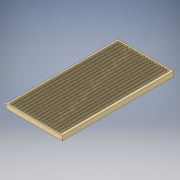
# Autodesk Inventor part: Lathhouse roof
Saved by Autodesk Inventor 2018 (Build 220112000, 112)
## iProperties
Created: 2019-05-09
Part Number: Lathhouse roof
Material: Generic
Document SubType Name: Modeling
Designer: 10043883
Density: 1 g/cm^3
Appearance: Wheat
Author: 10043883
Autodesk Inventor part; units mm, degrees
ref_plane "YZ Plane" through (0, 0, 0) normal (1, 0, 0) x (0, 1, 0)
ref_plane "XZ Plane" through (0, 0, 0) normal (0, 1, 0) x (-1, 0, 0)
ref_plane "XY Plane" through (0, 0, 0) normal (0, 0, 1) x (1, 0, 0)
sketch "Sketch1" plane through (0, 0, 0) normal (0, 1, 0) x (-1, 0, 0)
  line L0 (0, 0) -> (-3048, 0)
  line L1 (-3048, 0) -> (-3048, -6096)
  line L2 (-3048, -6096) -> (0, -6096)
  line L3 (0, -6096) -> (0, 0)
  dimension "d0" = 3048
  dimension "d1" = 6096
  constraints: 8 end point, 2 parallel, 1 horizontal, 1 perpendicular
  measures "d0" distance of L2.end L1.end
  measures "d1" distance of L1.end L0.end
extrude "Extrusion1" add sketch "Sketch1" along normal blind 254
sketch "Sketch2" plane through (0, 254, 0) normal (0, 1, 0) x (1, 0, 0)
  point P0 (0, 0)
sketch "Sketch3" plane through (0, 254, 0) normal (0, 1, 0) x (1, 0, 0)
  line L0 (94.7299, 6010.3245) -> (249.433, 6010.3245)
  line L1 (249.433, 6010.3245) -> (249.433, 63.9243)
  line L2 (249.433, 63.9243) -> (94.7299, 63.9243)
  line L3 (94.7299, 63.9243) -> (94.7299, 6010.3245)
  line L4 (427.233, 6010.3245) -> (427.233, 63.9243)
  line L5 (272.5299, 63.9243) -> (272.5299, 6010.3245)
  line L6 (427.233, 63.9243) -> (272.5299, 63.9243)
  line L7 (272.5299, 6010.3245) -> (427.233, 6010.3245)
  line L8 (605.033, 6010.3245) -> (605.033, 63.9243)
  line L9 (450.3299, 63.9243) -> (450.3299, 6010.3245)
  line L10 (605.033, 63.9243) -> (450.3299, 63.9243)
  line L11 (450.3299, 6010.3245) -> (605.033, 6010.3245)
  line L12 (782.833, 6010.3245) -> (782.833, 63.9243)
  line L13 (628.1299, 63.9243) -> (628.1299, 6010.3245)
  line L14 (782.833, 63.9243) -> (628.1299, 63.9243)
  line L15 (628.1299, 6010.3245) -> (782.833, 6010.3245)
  line L16 (960.633, 6010.3245) -> (960.633, 63.9243)
  line L17 (805.9299, 63.9243) -> (805.9299, 6010.3245)
  line L18 (960.633, 63.9243) -> (805.9299, 63.9243)
  line L19 (805.9299, 6010.3245) -> (960.633, 6010.3245)
  line L20 (1138.433, 6010.3245) -> (1138.433, 63.9243)
  line L21 (983.7299, 63.9243) -> (983.7299, 6010.3245)
  line L22 (1138.433, 63.9243) -> (983.7299, 63.9243)
  line L23 (983.7299, 6010.3245) -> (1138.433, 6010.3245)
  line L24 (1316.233, 6010.3245) -> (1316.233, 63.9243)
  line L25 (1161.5299, 63.9243) -> (1161.5299, 6010.3245)
  line L26 (1316.233, 63.9243) -> (1161.5299, 63.9243)
  line L27 (1161.5299, 6010.3245) -> (1316.233, 6010.3245)
  line L28 (1494.033, 6010.3245) -> (1494.033, 63.9243)
  line L29 (1339.3299, 63.9243) -> (1339.3299, 6010.3245)
  line L30 (1494.033, 63.9243) -> (1339.3299, 63.9243)
  line L31 (1339.3299, 6010.3245) -> (1494.033, 6010.3245)
  line L32 (1671.833, 6010.3245) -> (1671.833, 63.9243)
  line L33 (1517.1299, 63.9243) -> (1517.1299, 6010.3245)
  line L34 (1671.833, 63.9243) -> (1517.1299, 63.9243)
  line L35 (1517.1299, 6010.3245) -> (1671.833, 6010.3245)
  line L36 (1849.633, 6010.3245) -> (1849.633, 63.9243)
  line L37 (1694.9299, 63.9243) -> (1694.9299, 6010.3245)
  line L38 (1849.633, 63.9243) -> (1694.9299, 63.9243)
  line L39 (1694.9299, 6010.3245) -> (1849.633, 6010.3245)
  line L40 (2027.433, 6010.3245) -> (2027.433, 63.9243)
  line L41 (1872.7299, 63.9243) -> (1872.7299, 6010.3245)
  line L42 (2027.433, 63.9243) -> (1872.7299, 63.9243)
  line L43 (1872.7299, 6010.3245) -> (2027.433, 6010.3245)
  line L44 (2205.233, 6010.3245) -> (2205.233, 63.9243)
  line L45 (2050.5299, 63.9243) -> (2050.5299, 6010.3245)
  line L46 (2205.233, 63.9243) -> (2050.5299, 63.9243)
  line L47 (2050.5299, 6010.3245) -> (2205.233, 6010.3245)
  line L48 (2383.033, 6010.3245) -> (2383.033, 63.9243)
  line L49 (2228.3299, 63.9243) -> (2228.3299, 6010.3245)
  line L50 (2383.033, 63.9243) -> (2228.3299, 63.9243)
  line L51 (2228.3299, 6010.3245) -> (2383.033, 6010.3245)
  line L52 (2560.833, 6010.3245) -> (2560.833, 63.9243)
  line L53 (2406.1299, 63.9243) -> (2406.1299, 6010.3245)
  line L54 (2560.833, 63.9243) -> (2406.1299, 63.9243)
  line L55 (2406.1299, 6010.3245) -> (2560.833, 6010.3245)
  line L56 (2738.633, 6010.3245) -> (2738.633, 63.9243)
  line L57 (2583.9299, 63.9243) -> (2583.9299, 6010.3245)
  line L58 (2738.633, 63.9243) -> (2583.9299, 63.9243)
  line L59 (2583.9299, 6010.3245) -> (2738.633, 6010.3245)
  line L60 (2916.433, 6010.3245) -> (2916.433, 63.9243)
  line L61 (2761.7299, 63.9243) -> (2761.7299, 6010.3245)
  line L62 (2916.433, 63.9243) -> (2761.7299, 63.9243)
  line L63 (2761.7299, 6010.3245) -> (2916.433, 6010.3245)
  point P0 (0, 0)
  dimension "d6" = 177.8
  constraints: 128 end point, 2 horizontal, 2 parallel, 1 collinear, 1 perpendicular, 119 other
  measures "d6" distance of L0.end L4.start
extrude "Extrusion2" cut sketch "Sketch3" against normal through all
body "Solid1"
